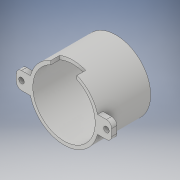
# Autodesk Inventor part: 音箱
Saved by Autodesk Inventor 2019 (Build 230136000, 136)
## iProperties
Created: 2020-10-10
Part Number: 音箱
Material: 一般
Document SubType Name: Modeling
Designer: Owner
Density: 1 g/cm^3
Appearance: 預設
Author: Owner
Autodesk Inventor part; units mm, degrees
ref_plane "YZ Plane" through (0, 0, 0) normal (1, 0, 0) x (0, 1, 0)
ref_plane "XZ Plane" through (0, 0, 0) normal (0, 1, 0) x (-1, 0, 0)
ref_plane "XY Plane" through (0, 0, 0) normal (0, 0, 1) x (1, 0, 0)
sketch "草圖1" plane through (0, 0, 0) normal (0, 0, 1) x (1, 0, 0)
  circle A0 centre (0, 0) radius 20
  dimension "d0" = 40
  constraints: 1 centre point, 1 coincident
  measures "d0" diameter of A0
extrude "擠出1" add sketch "草圖1" along normal blind 30
sketch "草圖2" plane through (0, 0, 30) normal (0, 0, 1) x (1, 0, 0)
  circle A0 centre (0, 0) radius 18
  circle A1 centre (0, 0) radius 20 projected
  dimension "d3" = 2
  constraints: 1 centre point, 1 coincident
  measures "d3" radial gap between concentric circles of A1 A0
extrude "擠出2" cut sketch "草圖2" against normal blind 28 contours A0
sketch "草圖3" plane through (0, 0, 30) normal (0, 0, 1) x (1, 0, 0)
  line L0 (-7.5, 20) -> (7.5, 20)
  line L1 (7.5, 20) -> (7.5, 10)
  line L2 (7.5, 10) -> (-7.5, 10)
  line L3 (-7.5, 10) -> (-7.5, 20)
  circle A0 centre (0, 0) radius 20 projected
  point P0 (0, 20)
  dimension "d6" = 15
  dimension "d7" = 10
  constraints: 8 end point, 2 parallel, 1 horizontal, 1 midpoint, 1 perpendicular, 1 tangent, 1 vertical alignment
  measures "d6" distance of L0.start L0.end
  measures "d7" distance of L2.end L0.start
extrude "擠出3" cut sketch "草圖3" against normal blind 5 contours L0 A0 L3 | L0 L1 A0 | A0 L1 L2 L3 picked at (0, 13.3333)
sketch "草圖4" plane through (0, 0, 30) normal (0, 0, 1) x (1, 0, 0)
  line L0 (-27.5, -5) -> (27.5, -5)
  line L1 (27.5, -5) -> (27.5, 5)
  line L2 (27.5, 5) -> (-27.5, 5)
  line L3 (-27.5, 5) -> (-27.5, -5)
  point P0 (0, 0)
  point P1 (0, -5)
  point P2 (-27.5, 0)
  dimension "d10" = 10
  dimension "d11" = 55
  constraints: 8 end point, 2 midpoint, 2 parallel, 1 horizontal, 1 horizontal alignment, 1 perpendicular, 1 vertical alignment
  measures "d10" distance of L2.end L0.start
  measures "d11" distance of L0.start L0.end
extrude "擠出4" add sketch "草圖4" against normal blind 3
sketch "草圖5" plane through (0, 0, 30) normal (0, 0, 1) x (1, 0, 0)
  circle A0 centre (0, 0) radius 18
  arc A1 (-17.2916, -5) -> (17.2916, -5) centre (0, 0) ccw projected
  dimension "d14" = 0
  constraints: 1 centre point, 1 coincident
  measures "d14" radial gap between concentric circles of A1 A0
extrude "擠出5" cut sketch "草圖5" against normal up to surface (28 mm away)
sketch "草圖6" plane through (0, 0, 27) normal (0, 0, -1) x (-1, 0, 0)
  circle A0 centre (-24.5, 0) radius 1.6
  line L0 (-27.5, 5) -> (-27.5, -5) projected
  point P0 (0, 0)
  dimension "d17" = 3.2
  dimension "d18" = 3
  constraints: 1 centre point
  measures "d17" diameter of A0
  measures "d18" distance from line of L0 A0.centre
extrude "擠出6" cut sketch "草圖6" against normal up to surface (3 mm away)
mirror "鏡射1" about plane through (0, 0, 0) normal (1, 0, 0) of "擠出6"
fillet "圓角1" radius 3 4 edges at (27.5, 5, 28.5) (27.5, -5, 28.5) (-27.5, 5, 28.5) (-27.5, -5, 28.5)
